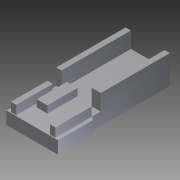
# Autodesk Inventor part: fio
Saved by Autodesk Inventor 2012 (Build 160160000, 160)
## iProperties
Created: 2012-12-27
Part Number: fio
Material: Default
Document SubType Name: Modeling
Designer: otrebor
Density: 1 g/cm^3
Author: otrebor
Autodesk Inventor part; units mm, degrees
ref_plane "YZ Plane" through (0, 0, 0) normal (1, 0, 0) x (0, 1, 0)
ref_plane "XZ Plane" through (0, 0, 0) normal (0, 1, 0) x (-1, 0, 0)
ref_plane "XY Plane" through (0, 0, 0) normal (0, 0, 1) x (1, 0, 0)
sketch "Boceto1" plane through (0, 0, 0) normal (0, 0, 1) x (1, 0, 0)
  line L0 (0, 0) -> (0, 19.566)
  line L1 (2, 65) -> (2, 21)
  line L2 (2, 21) -> (0, 19.566)
  line L3 (2, 65) -> (14.5, 65)
  line L4 (29, 0) -> (29, 19.566)
  line L5 (27, 65) -> (27, 21)
  line L6 (27, 21) -> (29, 19.566)
  line L7 (27, 65) -> (14.5, 65)
  line L8 (0, 0) -> (29, 0)
  constraints: 18 end point, 2 perpendicular, 1 parallel, 1 vertical
extrude "Extrusión1" add sketch "Boceto1" along normal blind 7
sketch "Boceto2" plane through (0, 0, 7) normal (0, 0, 1) x (1, 0, 0)
  line L0 (27, 65) -> (27, 21) projected
  line L1 (2, 65) -> (27, 65) projected
  line L2 (2, 21) -> (2, 65) projected
  line L3 (2, 65) -> (5, 65)
  line L4 (2, 65) -> (2, 26)
  line L5 (5, 26) -> (5, 65)
  line L6 (27, 65) -> (24, 65)
  line L7 (24, 65) -> (24, 41)
  line L8 (27, 65) -> (27, 26)
  line L9 (5, 26) -> (2, 26)
  line L10 (24, 26) -> (27, 26)
  line L11 (24.1227, 26) -> (22, 26)
  line L12 (22, 26) -> (22, 41)
  line L13 (22, 41) -> (24, 41)
  dimension "d7" = 15
  constraints: 22 end point, 5 perpendicular, 2 collinear, 2 point on line, 1 parallel
  measures "d7" distance of L11.end L12.end
extrude "Extrusión2" add sketch "Boceto2" along normal blind 9
sketch "Boceto3" plane through (0, 0, 7) normal (0, 0, 1) x (1, 0, 0)
  line L0 (5, 65) -> (24, 65) projected
  line L1 (29, 0) -> (0, 0) projected
  line L2 (22, 41) -> (24, 41) projected
  line L3 (2, 0.5) -> (2, 21)
  line L4 (2, 21) -> (5, 21)
  line L5 (5, 21) -> (5, 0.5)
  line L6 (5, 0.5) -> (2, 0.5)
  line L7 (27, 0.5) -> (27, 21)
  line L8 (27, 21) -> (24, 21)
  line L9 (24, 21) -> (24, 0.5)
  line L10 (24, 0.5) -> (27, 0.5)
  dimension "d9" = 20.5
  constraints: 16 end point, 4 perpendicular, 1 parallel
  measures "d9" distance of L4.end L5.end
extrude "Extrusión3" add sketch "Boceto3" along normal blind 5
sketch "Boceto4" plane through (0, 0, 7) normal (0, 0, 1) x (1, 0, 0)
  line L0 (29, 0) -> (0, 0) projected
  line L1 (7, 10) -> (13, 10)
  line L2 (13, 10) -> (13, 27)
  line L3 (13, 27) -> (7, 27)
  line L4 (7, 27) -> (7, 10)
  constraints: 8 end point, 2 parallel, 1 perpendicular
extrude "Extrusión4" add sketch "Boceto4" along normal blind 4
